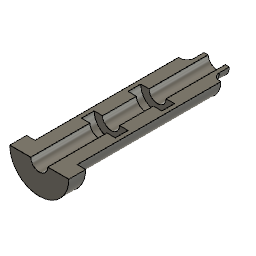
HalfAxle (Autodesk Fusion 360 design; units mm, degrees)
Autodesk Fusion 360 part; units mm, degrees
sketch "Sketch1" plane through (0, 0, 0) normal (0, 0, 1) x (1, 0, 0)
  circle A0 centre (0, 0) radius 2.5 construction
  line L0 (-2.5, 0) -> (2.5, 0) construction
  circle A1 centre (0, 0) radius 1.01 construction
  arc A2 (-2.5, 0) -> (2.5, 0) centre (0, 0) ccw
  arc A3 (-1.01, 0) -> (1.01, 0) centre (0, 0.0002) ccw
  line L1 (-2.5, 0) -> (-1.01, 0)
  line L2 (2.5, 0) -> (1.01, 0)
  dimension "d1" = 5
  dimension "d2" = 2.02
  constraint coincident A0.centre A1.centre
  constraint coincident A0 L0.start
  constraint coincident A0 L0.end
  constraint horizontal L0
  constraint midpoint A0.centre L0
  constraint coincident A1 A3.end
  constraint coincident L0 A3.end
  constraint coincident A1 A3.start
  constraint coincident L0 A3.start
  constraint equal A0 A2
  constraint equal A1 A3
  measures "d1" diameter of A0
  measures "d2" diameter of A1
extrude "Extrude1" add sketch "Sketch1" against normal blind 10.5
sketch "Sketch2" plane through (0, 0, 0) normal (0, 1, 0) x (1, 0, 0)
  line L0 (1.01, 3.5) -> (-1.01, 3.5) construction
  line L1 (-1.01, 3.5) -> (-1.01, 18.5) construction
  line L2 (-1.01, 18.5) -> (1.01, 18.5) construction
  line L3 (1.01, 18.5) -> (1.01, 3.5)
  line L4 (1.01, 3.5) -> (-1.01, 18.5) construction
  line L5 (-1.01, 3.5) -> (1.01, 18.5) construction
  line L6 (2, 2) -> (-2, 2) construction
  line L7 (-2, 2) -> (-2, 3.5) construction
  line L8 (-2, 3.5) -> (2, 3.5) construction
  line L9 (2, 3.5) -> (2, 2)
  line L10 (2, 2) -> (-2, 3.5) construction
  line L11 (-2, 2) -> (2, 3.5) construction
  line L12 (0, 2.75) -> (0, 3.5) construction
  line L13 (0, 0) -> (0, 2) construction
  line L14 (1.01, 0) -> (2.5, 0)
  line L15 (1.01, 10.5) -> (2.5, 10.5)
  line L16 (2, 3.5) -> (1.01, 3.5)
  line L17 (2, 2) -> (0, 2)
  line L18 (0, 2) -> (0, 18.5)
  line L19 (0, 18.5) -> (1.01, 18.5)
  point P0 (0, 11)
  point P1 (0, 2.75)
  dimension "d5" = 2.02
  dimension "d6" = 15
  dimension "d7" = 4
  dimension "d8" = 1.5
  dimension "d10" = 8
  constraint horizontal L0
  constraint perpendicular L0 L1
  constraint parallel L0 L2
  constraint parallel L1 L3
  constraint coincident L4 P0
  constraint coincident L5 P0
  constraint horizontal L6
  constraint perpendicular L6 L7
  constraint parallel L6 L8
  constraint parallel L7 L9
  constraint coincident L10 P1
  constraint coincident L11 P1
  constraint coincident P1 L12.start
  constraint midpoint L8 L12.end
  constraint midpoint L0 L12.end
  constraint coincident L13.start origin
  constraint vertical L13
  constraint midpoint L6 L13.end
  constraint midpoint L2 L18.end
  measures "d5" distance of L1.end L2.end
  measures "d6" distance of L0.end L1.end
  measures "d7" distance of L7.end L8.end
  measures "d8" distance of L6.end L7.end
  measures "d10" distance of L2 L15
revolve "Revolve1" cut sketch "Sketch2" angle 360 about axis through (0, 0, 1.75) along (0, 0, 1)
mirror "Mirror1" about plane through (0, 0, 0) normal (0, 0, 1) of bodies 1 merged
sketch "Sketch3" plane through (0, 0, 0) normal (0, 1, 0) x (1, 0, 0)
  line L0 (2.5, 8.5) -> (-2.5, 8.5) construction
  line L1 (-2.5, 8.5) -> (-2.5, -8.5) construction
  line L2 (-2.5, -8.5) -> (2.5, -8.5) construction
  line L3 (2.5, -8.5) -> (2.5, 8.5) construction
  line L4 (2.5, 8.5) -> (-2.5, -8.5) construction
  line L5 (-2.5, 8.5) -> (2.5, -8.5) construction
  line L6 (0, 0) -> (0, -8.5) construction
  line L7 (0, -8.5) -> (0, -4.25) construction
  point P0 (0, -4.25)
  dimension "d14" = 5
  dimension "d15" = 17
  constraint horizontal L0
  constraint perpendicular L0 L1
  constraint parallel L0 L2
  constraint parallel L1 L3
  constraint coincident L4 L6.start
  constraint coincident L5 L6.start
  constraint coincident L6.start origin
  constraint midpoint L2 L6.end
  constraint midpoint L6 P0
  constraint coincident P0 L7.end
  measures "d14" distance of L1.end L2.end
  measures "d15" distance of L0.end L1.end
sketch "Sketch4" plane through (0, 0, 10.5) normal (0, 0, 1) x (1, 0, 0)
  arc A0 (-1.01, 0) -> (1.01, 0) centre (0, 0) ccw
  line L0 (-1.01, 0) -> (-2.5, 0)
  arc A1 (-2.5, 0) -> (2.5, 0) centre (0, 0) ccw
  line L1 (2.5, 0) -> (1.01, 0)
  circle A2 centre (0, 0) radius 1.01 construction
  circle A3 centre (0, 0) radius 3.5 construction
  line L2 (-3.5, 0) -> (3.5, 0) construction
  arc A4 (-3.5, 0) -> (3.5, 0) centre (0, 0) ccw
  arc A5 (-1.01, 0) -> (1.01, 0) centre (0, 0) ccw
  line L3 (-3.5, 0) -> (-1.01, 0)
  line L4 (1.01, 0) -> (3.5, 0)
  dimension "d16" = 7
  constraint concentric A0 A2
  constraint coincident A0.end A2
  constraint concentric A0 A3
  constraint coincident A3 L2.start
  constraint coincident A3 L2.end
  constraint parallel L1 L2
  constraint midpoint A0.centre L2
  constraint coincident A0.end L1.end
  constraint coincident A0.start L0.start
  constraint equal A3 A4
  constraint coincident A0.centre A1.centre
  measures "d16" diameter of A3
extrude "Extrude2" add sketch "Sketch4" against normal up to surface (2 mm away) contours A1 A4 L3 L4
sketch "Sketch5" plane through (0, 0, -10.5) normal (0, 0, -1) x (-1, 0, 0)
  arc A0 (-1.01, 0) -> (1.01, 0) centre (0, 0) ccw construction
  line L0 (-1.01, 0) -> (-2.5, 0) construction
  arc A1 (-2.5, 0) -> (2.5, 0) centre (0, 0) ccw construction
  line L1 (2.5, 0) -> (1.01, 0) construction
  circle A2 centre (0, 0) radius 1.01 construction
  circle A3 centre (0, 0) radius 2.5 construction
  line L2 (-2.5, 0) -> (2.5, 0) construction
  circle A4 centre (0, 0) radius 1.5 construction
  arc A5 (-2.5, 0) -> (2.5, 0) centre (0, 0) ccw
  arc A6 (-1.5, 0) -> (1.5, 0) centre (0, 0) ccw
  line L3 (-2.5, 0) -> (-1.5, 0)
  line L4 (2.5, 0) -> (1.5, 0)
  dimension "d19" = -1
  constraint concentric A1 A2
  constraint coincident A0.end A2
  constraint concentric A2 A3
  constraint coincident A1.end A3
  constraint coincident L0.end A1.start
  constraint coincident A1.end L1.start
  constraint coincident L1 A6.end
  constraint coincident A4 A6.end
  constraint coincident L2 A6.start
  constraint coincident A4 A6.start
  constraint coincident A0.centre A1.centre
extrude "Extrude3" cut sketch "Sketch5" against normal up to surface (2 mm away)
fillet "Fillet1" radius 0.8 1 edges at (0, -1.5, -8.5)
equation "d2 = 2 mm * 1.01"
equation "d3 = -( ( 17 / 2 ) + 2 ) * 1 mm"
equation "d5 = 2 mm * 1.01"
